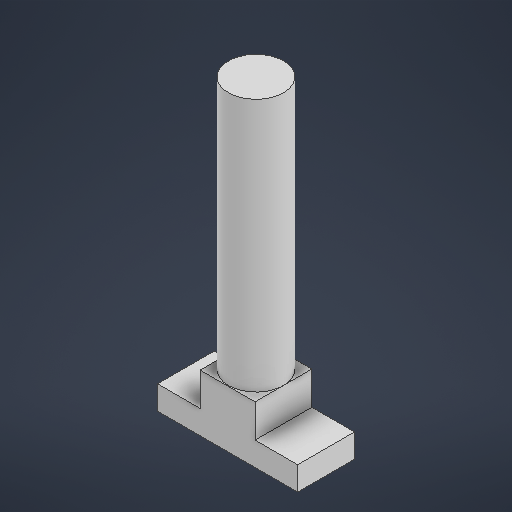
# Autodesk Inventor part: Press_Mandrel
Saved by Autodesk Inventor 2026.1 (Build 301233020, 233B)
## iProperties
Created: 2025-10-06
Part Number: Press_Mandrel
Material: Generic
Document SubType Name: Modeling
Designer: Gamec
Density: 1 g/cm^3
Appearance: Default
Author: Gamec
Autodesk Inventor part; units mm, degrees
ref_plane "YZ Plane" through (0, 0, 0) normal (1, 0, 0) x (0, 1, 0)
ref_plane "XZ Plane" through (0, 0, 0) normal (0, 1, 0) x (-1, 0, 0)
ref_plane "XY Plane" through (0, 0, 0) normal (0, 0, 1) x (1, 0, 0)
sketch "Sketch1" plane through (0, 0, 0) normal (0, 1, 0) x (-1, 0, 0)
  line L0 (-9.398, 3.81) -> (9.398, 3.81)
  line L1 (9.398, 3.81) -> (9.398, -3.81)
  line L2 (9.398, -3.81) -> (-9.398, -3.81)
  line L3 (-9.398, -3.81) -> (-9.398, 3.81)
  line L4 (-9.398, 3.81) -> (9.398, -3.81) construction
  line L5 (9.398, 3.81) -> (-9.398, -3.81) construction
  point P0 (0, 0)
  dimension "d0" = 18.796
  dimension "d1" = 7.62
  constraints: 12 end point, 2 midpoint, 2 parallel, 1 horizontal, 1 perpendicular
  measures "d0" distance of L1.end L2.end
  measures "d1" distance of L0.end L1.end
extrude "Extrusion1" add sketch "Sketch1" along normal blind 3.175
sketch "Sketch2" plane through (0, 3.175, 0) normal (0, 1, 0) x (1, 0, 0)
  line L0 (-9.398, -3.81) -> (9.398, -3.81) projected
  line L1 (3.683, 3.81) -> (-3.683, 3.81)
  line L2 (-3.683, 3.81) -> (-3.683, -3.81)
  line L3 (-3.683, -3.81) -> (3.683, -3.81)
  line L4 (3.683, -3.81) -> (3.683, 3.81)
  line L5 (3.683, 3.81) -> (-3.683, -3.81) construction
  line L6 (-3.683, 3.81) -> (3.683, -3.81) construction
  point P0 (0, 0)
  dimension "d4" = 7.366
  constraints: 12 end point, 2 midpoint, 2 parallel, 1 horizontal, 1 perpendicular, 1 point on line
  measures "d4" distance of L3.end L2.end
extrude "Extrusion2" add sketch "Sketch2" along normal blind 4.445
sketch "Sketch3" plane through (0, 7.62, 0) normal (0, 1, 0) x (1, 0, 0)
  circle A0 centre (0, 0) radius 3.7
  dimension "d7" = 7.4
  constraints: 1 centre point, 1 coincident
  measures "d7" diameter of A0
extrude "Extrusion3" add sketch "Sketch3" along normal blind 34
body "Solid1"
